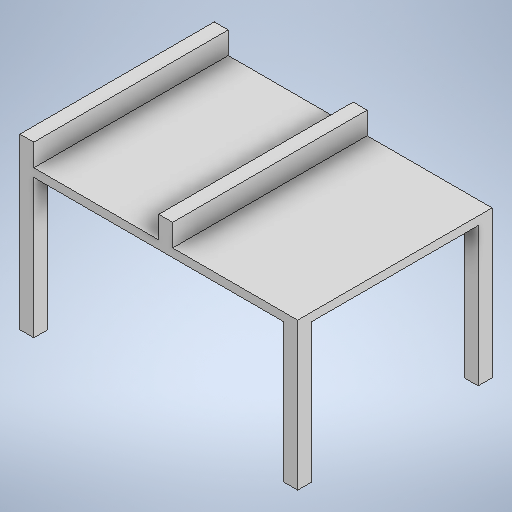
# Autodesk Inventor part: Table_2
Saved by Autodesk Inventor 2025 (Build 290162000, 162)
## iProperties
Created: 2024-07-31
Part Number: Table_2
Material: Generic
Document SubType Name: Modeling
Designer: User
Density: 1 g/cm^3
Appearance: Default
Author: User
Autodesk Inventor part; units mm, degrees
ref_plane "YZ Plane" through (0, 0, 0) normal (1, 0, 0) x (0, 1, 0)
ref_plane "XZ Plane" through (0, 0, 0) normal (0, 1, 0) x (-1, 0, 0)
ref_plane "XY Plane" through (0, 0, 0) normal (0, 0, 1) x (1, 0, 0)
sketch "Sketch1" plane through (0, 0, 0) normal (0, 1, 0) x (-1, 0, 0)
  line L0 (-500, 350) -> (500, 350)
  line L1 (500, 350) -> (500, -350)
  line L2 (500, -350) -> (-500, -350)
  line L3 (-500, -350) -> (-500, 350)
  line L4 (-500, 350) -> (500, -350) construction
  line L5 (500, 350) -> (-500, -350) construction
  line L6 (500, -350) -> (-50, -350)
  line L7 (-50, -350) -> (-50, 350)
  line L8 (-50, 350) -> (500, 350)
  line L9 (500, 350) -> (500, -350)
  line L10 (500, -350) -> (450, -350)
  line L11 (450, -350) -> (450, 350)
  line L12 (450, 350) -> (500, 350)
  line L13 (500, 350) -> (500, -350)
  line L14 (0, -350) -> (-50, -350)
  line L15 (-50, -350) -> (-50, 350)
  line L16 (-50, 350) -> (0, 350)
  line L17 (0, 350) -> (0, -350)
  point P0 (0, 0)
  point P1 (450, 350)
  dimension "d0" = 1000
  dimension "d1" = 700
  dimension "d2" = 550
  dimension "d3" = 50
  dimension "d4" = 50
  constraints: 36 end point, 8 parallel, 4 horizontal, 4 perpendicular, 3 point on line, 2 midpoint
  measures "d0" distance of L1.end L2.end
  measures "d1" distance of L0.end L1.end
  measures "d2" distance between parallel lines of L7 L1
  measures "d3" distance between parallel lines of L1 L11
  measures "d4" distance between parallel lines of L7 L17
extrude "Extrusion1" add sketch "Sketch1" along normal blind 110 contours L0 L17 L2 L7 | L0 L1 L2 L11
extrude "Extrusion2" add sketch "Sketch1" along normal blind 30 contours L0 L7 L2 L3 | L0 L11 L2 L17
sketch "Sketch2" plane through (0, 0, 0) normal (0, -1, 0) x (1, 0, 0)
  line L0 (500, -350) -> (50, -350) projected
  line L1 (500, -350) -> (450, -350)
  line L2 (450, -350) -> (450, -300)
  line L3 (450, -300) -> (500, -300)
  line L4 (500, -300) -> (500, -350)
  line L5 (50, 350) -> (500, 350) projected
  line L6 (500, 300) -> (450, 300)
  line L7 (450, 300) -> (450, 350)
  line L8 (450, 350) -> (500, 350)
  line L9 (500, 350) -> (500, 300)
  line L10 (-500, -350) -> (-500, 350) projected
  line L11 (-500, -350) -> (-450, -350)
  line L12 (-450, -350) -> (-450, -300)
  line L13 (-450, -300) -> (-500, -300)
  line L14 (-500, -300) -> (-500, -350)
  line L15 (-500, 350) -> (-450, 350)
  line L16 (-450, 350) -> (-450, 300)
  line L17 (-450, 300) -> (-500, 300)
  line L18 (-500, 300) -> (-500, 350)
  point P0 (0, 0)
  dimension "d9" = 50
  dimension "d10" = 50
  dimension "d11" = 50
  dimension "d12" = 50
  dimension "d13" = 50
  dimension "d14" = 50
  dimension "d15" = 50
  dimension "d16" = 50
  constraints: 32 end point, 8 parallel, 4 horizontal, 4 perpendicular, 2 point on line
  measures "d9" distance of L1.end L2.end
  measures "d10" distance of L2.end L3.end
  measures "d11" distance of L6.start L6.end
  measures "d12" distance of L6.end L7.end
  measures "d13" distance of L15.end L16.end
  measures "d14" distance of L16.end L17.end
  measures "d15" distance of L12.end L13.end
  measures "d16" distance of L11.end L12.end
extrude "Extrusion3" add sketch "Sketch2" along normal blind 500
body "Solid1"
